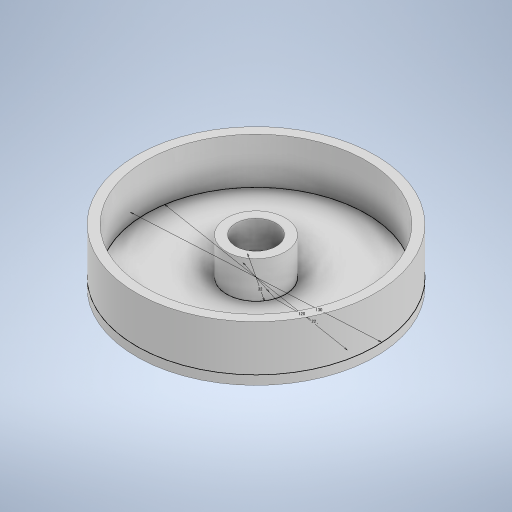
# Autodesk Inventor part: tire out130 in 22 5mm inward
Saved by Autodesk Inventor 2023 (Build 270158000, 158)
## iProperties
Created: 2022-11-06
Part Number: tire out130 in 22 5mm inward
Material: 一般
Document SubType Name: Modeling
Designer: RM206user
Density: 1 g/cm^3
Appearance: 既定
Author: RM206user
Autodesk Inventor part; units mm, degrees
ref_plane "YZ Plane" through (0, 0, 0) normal (1, 0, 0) x (0, 1, 0)
ref_plane "XZ Plane" through (0, 0, 0) normal (0, 1, 0) x (-1, 0, 0)
ref_plane "XY Plane" through (0, 0, 0) normal (0, 0, 1) x (1, 0, 0)
sketch "スケッチ1" plane through (0, 0, 0) normal (0, 1, 0) x (-1, 0, 0)
  circle A0 centre (0, 0) radius 65
  circle A1 centre (0, 0) radius 60
  circle A2 centre (0, 0) radius 11
  circle A3 centre (0, 0) radius 16
  dimension "d0" = 130
  dimension "d1" = 120
  dimension "d2" = 22
  dimension "d3" = 32
  constraints: 4 centre point, 4 coincident
  measures "d0" diameter of A0
  measures "d1" diameter of A1
  measures "d2" diameter of A2
  measures "d3" diameter of A3
extrude "押し出し1" add sketch "スケッチ1" against normal blind 5 contours A0 | A1 | A2 | A3
extrude "押し出し2" add sketch "スケッチ1" along normal blind 20 contours A3
extrude "押し出し3" add sketch "スケッチ1" along normal blind 25 contours A0
extrude "押し出し5" add sketch "スケッチ1" along normal blind 5 contours A2
sketch "スケッチ3" plane through (0, 5, 0) normal (0, 1, 0) x (1, 0, 0)
  circle A0 centre (0, 0) radius 2.5
  dimension "d15" = 5
  constraints: 1 centre point, 1 coincident
  measures "d15" diameter of A0
extrude "押し出し6" cut sketch "スケッチ3" against normal blind 2
sketch "スケッチ4" plane through (0, -5, 0) normal (0, -1, 0) x (1, 0, 0)
  circle A0 centre (0, 0) radius 60 projected
  circle A1 centre (0, 0) radius 16 projected
  circle A2 centre (0, 0) radius 11 projected
  circle A3 centre (0, 0) radius 2.5 projected
